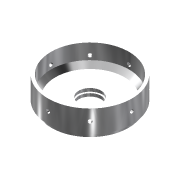
# Autodesk Inventor part: Forward Bulkhead
Saved by Autodesk Inventor 2016 SP1 (Build 200210100, 210)
## iProperties
Created: 2015-12-03
Part Number: Forward Bulkhead
Material: Aluminum 6061 T6 0 Cold Formed
Document SubType Name: Modeling
Designer: Jared
Density: 2.7 g/cm^3
Appearance: Aluminum - Flat
Author: Jared
Autodesk Inventor part; units mm, degrees
ref_plane "YZ Plane" through (0, 0, 0) normal (1, 0, 0) x (0, 1, 0)
ref_plane "XZ Plane" through (0, 0, 0) normal (0, 1, 0) x (-1, 0, 0)
ref_plane "XY Plane" through (0, 0, 0) normal (0, 0, 1) x (1, 0, 0)
sketch "Sketch1" plane through (0, 0, 0) normal (0, 0, 1) x (1, 0, 0)
  line L0 (-89.2439, 56.3562) -> (-82.8939, 56.3562)
  line L1 (-23.7723, -1.5875) -> (-23.7723, 4.7625)
  line L2 (-23.7723, 4.7625) -> (-27.5108, 4.7625)
  line L3 (-27.5108, 4.7625) -> (-27.5108, 9.1757)
  line L4 (-27.5108, 9.1757) -> (-23.7723, 9.1757)
  line L5 (-23.7723, -1.5875) -> (-23.7723, 4.7625)
  line L6 (-23.7723, 9.1757) -> (-23.7723, 14.2875)
  line L7 (0.0529, 0) -> (0.0529, 21.3316)
  line L8 (-89.2439, 8.7313) -> (-81.8144, 8.7312)
  line L9 (-81.8144, 8.7312) -> (-81.8144, 0)
  line L10 (-89.2439, 56.3562) -> (-89.2439, 8.7313)
  line L11 (-81.8144, 0) -> (-81.8144, -1.5875)
  line L12 (-81.8144, -1.5875) -> (-23.7723, -1.5875)
  line L13 (-23.7723, -1.5875) -> (-23.7723, -1.5875)
  line L14 (-82.8939, 23.8125) -> (-73.3689, 14.2875)
  line L15 (-82.8939, 56.3562) -> (-82.8939, 23.8125)
  line L16 (-73.3689, 14.2875) -> (-23.7723, 14.2875)
  point P0 (0, 0)
  dimension "d3" = 23.8252
  dimension "d8" = 15.875
  dimension "d9" = 6.35
  dimension "d10" = 3.7386
  dimension "d11" = 4.4132
  dimension "d12" = 5.1117
  dimension "d26" = 7.4295
  dimension "d28" = 1.5875
  dimension "d29" = 8.7312
  dimension "d30" = 47.625
  dimension "d31" = 58.0422
  dimension "d32" = 1.5875
  dimension "d35" = 49.5967
  dimension "d37" = 135
  dimension "d40" = 89.2969
  dimension "d41" = 25.4
  dimension "d42" = 32.5438
  dimension "d51" = 6.35
  constraints: 34 end point, 10 perpendicular, 3 vertical, 1 horizontal, 1 parallel
  measures "d3" distance of point (0, 0) L1.start
  measures "d8" distance of L1.start L6.end
  measures "d9" distance of L1.start L1.end
  measures "d10" distance of L1.end L2.end
  measures "d11" distance of L2.end L3.end
  measures "d12" distance of L4.end L6.end
  measures "d26" distance of L8.start L8.end
  measures "d28" distance of L9.end L11.end
  measures "d29" distance of L8.end L9.end
  measures "d30" distance of L0.start L8.start
  measures "d31" distance of L11.end L12.end
  measures "d32" distance from line of point (0, 0) L12
  measures "d35" distance of L14.end L6.end
  measures "d37" angle of L16 L14
  measures "d40" distance between parallel lines of L7 L10
  measures "d41" distance from line of L14.start L12
  measures "d42" distance of L0.end L14.start
  measures "d51" distance of L0.start L0.end
revolve "Revolution3" add sketch "Sketch1" angle 360 about axis through (0.0529, 0, 0) along (0, 1, 0)
sketch "Sketch2" plane through (0, 0, 0) normal (1, 0, 0) x (0, 1, 0)
  line L0 (56.3562, -82.9469) -> (56.3562, 82.9469) projected
  circle A0 centre (32.5818, 0) radius 3.9688
  line L1 (56.3562, 0) -> (32.5818, 0)
  point P0 (0, 0)
  dimension "d45" = 7.9375
  dimension "d53" = 23.7744
  constraints: 2 end point, 1 centre point, 1 horizontal, 1 midpoint
  measures "d45" diameter of A0
  measures "d53" distance of L1.start L1.end
extrude "Extrusion1" cut sketch "Sketch2" along normal blind 207.9625
pattern_circular "Circular Pattern1" count 8 over 360 about axis through (0.0529, 40.0844, 0) along (0, 1, 0) of "Extrusion1"
body "Solid3"
